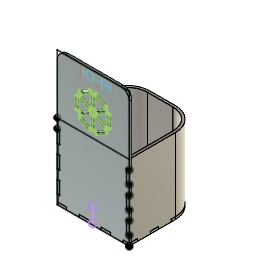
porta_lapices_v1 (Autodesk Fusion 360 design; units mm, degrees)
Autodesk Fusion 360 part; units mm, degrees
(part 1 of 3)
sketch "Boceto1" plane through (0, 0, 0) normal (0, 0, 1) x (1, 0, 0)
  line L0 (15, 40) -> (-15, 40)
  line L1 (-40, 15) -> (-40, -40)
  line L2 (40, -40) -> (40, 15)
  line L3 (40, 40) -> (-40, -40) construction
  line L4 (-40, 40) -> (40, -40) construction
  arc A0 (-15, 40) -> (-40, 15) centre (-15, 15) ccw
  line L5 (43, -40) -> (43, 15)
  line L6 (15, 43) -> (-15, 43)
  arc A1 (-15, 43) -> (-43, 15) centre (-15, 15) ccw
  line L7 (-43, 15) -> (-43, -40)
  line L8 (-40, -40) -> (-43, -40)
  line L9 (40, -40) -> (43, -40)
  arc A2 (40, 15) -> (15, 40) centre (15, 15) ccw
  arc A3 (43, 15) -> (15, 43) centre (15, 15) ccw
  dimension "d1" = 80
  dimension "d2" = 80
  dimension "d3" = 25
  dimension "d32" = 25
  dimension "d33" = 28
  constraint horizontal L0
  constraint perpendicular L0 L1
  constraint parallel L1 L2
  constraint coincident L3 origin
  constraint coincident L4 origin
  constraint coincident L4.start L1
  constraint coincident L4.start L0
  constraint tangent L1 A0
  constraint tangent L0 A0
  constraint coincident L3.start L0
  constraint coincident L3.start L2
  constraint perpendicular L7 L8
  constraint perpendicular L5 L9
  constraint concentric A0 A1
  constraint tangent A1 L7
  constraint tangent L6 A1
  constraint coincident L6 A1.end
  constraint tangent L2 A2
  constraint tangent L0 A2
  constraint tangent L5 A3
  constraint tangent L6 A3
  measures "d1" distance of L1.end L2.start
  measures "d2" distance of L4.start L1.end
  measures "d3" radius of A0
  measures "d32" radius of A2
  measures "d33" radius of A3
extrude "Extruir1" add sketch "Boceto1" along normal blind 90 makes body 1
sketch "Boceto5" plane through (0, -40, 0) normal (0, -1, 0) x (1, 0, 0)
  line L0 (-43, 0) -> (-40, 0)
  line L1 (-40, 0) -> (-40, 90)
  line L2 (-40, 90) -> (-43, 90)
  line L3 (-43, 90) -> (-43, 0)
  line L4 (-43, 90) -> (43, 90)
  line L5 (43, 90) -> (43, 0)
  line L6 (43, 0) -> (-43, 0)
  line L7 (-43, 0) -> (-43, 90)
  line L8 (-43, 78.75) -> (-40, 78.75)
  line L9 (-40, 78.75) -> (-40, 63.75)
  line L10 (-40, 63.75) -> (-43, 63.75)
  line L11 (-43, 63.75) -> (-43, 78.75)
  line L12 (-43, 52.5) -> (-40, 52.5)
  line L13 (-40, 52.5) -> (-40, 37.5)
  line L14 (-40, 37.5) -> (-43, 37.5)
  line L15 (-43, 37.5) -> (-43, 52.5)
  line L16 (-43, 26.25) -> (-40, 26.25)
  line L17 (-40, 26.25) -> (-40, 11.25)
  line L18 (-40, 11.25) -> (-43, 11.25)
  line L19 (-43, 11.25) -> (-43, 26.25)
  line L20 (-41.5, 78.75) -> (-41.5, 90) construction
  line L21 (-41.5, 63.75) -> (-41.5, 52.5) construction
  line L22 (-41.5, 37.5) -> (-41.5, 26.25) construction
  line L23 (-41.5, 11.25) -> (-41.5, 0) construction
  line L24 (0, 20) -> (0, 2.5)
  line L25 (43, 78.75) -> (40, 78.75)
  line L26 (40, 78.75) -> (40, 63.75)
  line L27 (40, 63.75) -> (43, 63.75)
  line L28 (40, 52.5) -> (40, 37.5)
  line L29 (43, 52.5) -> (40, 52.5)
  line L30 (40, 37.5) -> (43, 37.5)
  line L31 (43, 26.25) -> (40, 26.25)
  line L32 (40, 26.25) -> (40, 11.25)
  line L33 (40, 11.25) -> (43, 11.25)
  line L34 (-43, 160) -> (43, 160)
  line L35 (43, 160) -> (43, 90)
  line L36 (-43, 90) -> (-43, 160)
  line L37 (-4.7613, 96.0744) -> (-4.9442, 96.1341)
  line L38 (-4.9442, 96.1341) -> (-5.0659, 96.2025)
  spline S0 degree 3 poles (-5.0659, 96.2025) (-5.1328, 96.2402) (-7.6163, 97.6743) (-10.5848, 99.3893) knots 0 0 0 0 1 1 1 1
  line L39 (-10.5848, 99.3893) -> (-15.9822, 102.5077)
  line L40 (-15.9822, 102.5077) -> (-16.0924, 102.5916)
  spline S1 degree 3 poles (-16.0924, 102.5916) (-16.153, 102.6377) (-16.2592, 102.7361) (-16.3285, 102.8101) knots 0 0 0 0 1 1 1 1
  line L41 (-16.3285, 102.8101) -> (-16.4544, 102.9447)
  line L42 (-16.4544, 102.9447) -> (-16.5495, 103.1069)
  line L43 (-16.5495, 103.1069) -> (-16.6447, 103.269)
  line L44 (-16.6447, 103.269) -> (-16.7101, 103.4685)
  line L45 (-16.7101, 103.4685) -> (-16.7754, 103.6681)
  line L46 (-16.7754, 103.6681) -> (-16.785, 103.9516)
  line L47 (-16.785, 103.9516) -> (-16.7946, 104.2351)
  line L48 (-16.7946, 104.2351) -> (-16.7633, 104.3825)
  spline S2 degree 3 poles (-16.7633, 104.3825) (-16.7461, 104.4635) (-16.7028, 104.6053) (-16.6672, 104.6975) knots 0 0 0 0 1 1 1 1
  line L49 (-16.6672, 104.6975) -> (-16.6024, 104.8651)
  line L50 (-16.6024, 104.8651) -> (-16.5142, 104.9997)
  spline S3 degree 3 poles (-16.5142, 104.9997) (-16.4658, 105.0737) (-16.3697, 105.1945) (-16.3008, 105.2682) knots 0 0 0 0 1 1 1 1
  line L51 (-16.3008, 105.2682) -> (-16.1755, 105.4021)
  line L52 (-16.1755, 105.4021) -> (-15.999, 105.5196)
  line L53 (-15.999, 105.5196) -> (-15.8224, 105.637)
  line L54 (-15.8224, 105.637) -> (-15.6713, 105.6957)
  line L55 (-15.6713, 105.6957) -> (-15.5201, 105.7543)
  line L56 (-15.5201, 105.7543) -> (-15.343, 105.7902)
  line L57 (-15.343, 105.7902) -> (-15.1659, 105.8261)
  line L58 (-15.1659, 105.8261) -> (-14.9125, 105.8147)
  line L59 (-14.9125, 105.8147) -> (-14.6591, 105.8034)
  line L60 (-14.6591, 105.8034) -> (-14.5052, 105.759)
  line L61 (-14.5052, 105.759) -> (-14.3513, 105.7146)
  line L62 (-14.3513, 105.7146) -> (-14.2217, 105.6493)
  spline S4 degree 3 poles (-14.2217, 105.6493) (-14.1504, 105.6134) (-11.6538, 104.1758) (-8.6737, 102.4548) knots 0 0 0 0 1 1 1 1
  line L63 (-8.6737, 102.4548) -> (-3.2554, 99.3256)
  line L64 (-3.2554, 99.3256) -> (-3.0994, 99.2079)
  line L65 (-3.0994, 99.2079) -> (-2.9434, 99.0901)
  line L66 (-2.9434, 99.0901) -> (-2.8301, 98.9534)
  spline S5 degree 3 poles (-2.8301, 98.9534) (-2.6895, 98.7838) (-2.5801, 98.5915) (-2.5074, 98.3861) knots 0 0 0 0 1 1 1 1
  line L67 (-2.5074, 98.3861) -> (-2.4515, 98.2285)
  line L68 (-2.4515, 98.2285) -> (-2.4252, 98.0654)
  line L69 (-2.4252, 98.0654) -> (-2.3989, 97.9023)
  line L70 (-2.3989, 97.9023) -> (-2.4109, 97.677)
  line L71 (-2.4109, 97.677) -> (-2.4228, 97.4517)
  line L72 (-2.4228, 97.4517) -> (-2.4668, 97.298)
  line L73 (-2.4668, 97.298) -> (-2.5107, 97.1444)
  line L74 (-2.5107, 97.1444) -> (-2.5919, 96.983)
  line L75 (-2.5919, 96.983) -> (-2.6731, 96.8216)
  line L76 (-2.6731, 96.8216) -> (-2.7709, 96.6914)
  spline S6 degree 3 poles (-2.7709, 96.6914) (-2.9905, 96.3994) (-3.3229, 96.1708) (-3.6934, 96.0572) knots 0 0 0 0 1 1 1 1
  line L77 (-3.6934, 96.0572) -> (-3.8373, 96.0131)
  line L78 (-3.8373, 96.0131) -> (-4.2079, 96.0139)
  line L79 (-4.2079, 96.0139) -> (-4.5785, 96.0147)
  line L80 (-4.5785, 96.0147) -> (-4.7613, 96.0744)
  spline S7 degree 3 poles (-3.947, 96.0562) (-3.6813, 96.1032) (-3.4436, 96.2003) (-3.2159, 96.3547) knots 0 0 0 0 1 1 1 1
  line L81 (-3.2159, 96.3547) -> (-3.0924, 96.4384)
  line L82 (-3.0924, 96.4384) -> (-2.9655, 96.567)
  line L83 (-2.9655, 96.567) -> (-2.8386, 96.6956)
  line L84 (-2.8386, 96.6956) -> (-2.7384, 96.8488)
  line L85 (-2.7384, 96.8488) -> (-2.6382, 97.0019)
  line L86 (-2.6382, 97.0019) -> (-2.5742, 97.1678)
  line L87 (-2.5742, 97.1678) -> (-2.5102, 97.3337)
  line L88 (-2.5102, 97.3337) -> (-2.4764, 97.5292)
  line L89 (-2.4764, 97.5292) -> (-2.4425, 97.7247)
  line L90 (-2.4425, 97.7247) -> (-2.4568, 97.8898)
  line L91 (-2.4568, 97.8898) -> (-2.4711, 98.0549)
  line L92 (-2.4711, 98.0549) -> (-2.5105, 98.2052)
  spline S8 degree 3 poles (-2.5105, 98.2052) (-2.6122, 98.5936) (-2.8445, 98.9405) (-3.1621, 99.1785) knots 0 0 0 0 1 1 1 1
  line L93 (-3.1621, 99.1785) -> (-3.2764, 99.2641)
  line L94 (-3.2764, 99.2641) -> (-8.7367, 102.4202)
  line L95 (-8.7367, 102.4202) -> (-14.1971, 105.5763)
  line L96 (-14.1971, 105.5763) -> (-14.3653, 105.6451)
  line L97 (-14.3653, 105.6451) -> (-14.5336, 105.714)
  line L98 (-14.5336, 105.714) -> (-14.7328, 105.7486)
  line L99 (-14.7328, 105.7486) -> (-14.9321, 105.7832)
  line L100 (-14.9321, 105.7832) -> (-15.1074, 105.7692)
  line L101 (-15.1074, 105.7692) -> (-15.2826, 105.7552)
  line L102 (-15.2826, 105.7552) -> (-15.4644, 105.7025)
  line L103 (-15.4644, 105.7025) -> (-15.6461, 105.6499)
  line L104 (-15.6461, 105.6499) -> (-15.8042, 105.5658)
  line L105 (-15.8042, 105.5658) -> (-15.9623, 105.4816)
  line L106 (-15.9623, 105.4816) -> (-16.0977, 105.3723)
  line L107 (-16.0977, 105.3723) -> (-16.2331, 105.2631)
  line L108 (-16.2331, 105.2631) -> (-16.3447, 105.1271)
  line L109 (-16.3447, 105.1271) -> (-16.4563, 104.9911)
  line L110 (-16.4563, 104.9911) -> (-16.5586, 104.7811)
  line L111 (-16.5586, 104.7811) -> (-16.661, 104.5711)
  line L112 (-16.661, 104.5711) -> (-16.6955, 104.4346)
  line L113 (-16.6955, 104.4346) -> (-16.73, 104.2981)
  line L114 (-16.73, 104.2981) -> (-16.7415, 104.0986)
  line L115 (-16.7415, 104.0986) -> (-16.753, 103.8991)
  line L116 (-16.753, 103.8991) -> (-16.7101, 103.692)
  line L117 (-16.7101, 103.692) -> (-16.6671, 103.485)
  line L118 (-16.6671, 103.485) -> (-16.5626, 103.272)
  line L119 (-16.5626, 103.272) -> (-16.458, 103.059)
  line L120 (-16.458, 103.059) -> (-16.3418, 102.919)
  line L121 (-16.3418, 102.919) -> (-16.2256, 102.779)
  line L122 (-16.2256, 102.779) -> (-16.0999, 102.6775)
  line L123 (-16.0999, 102.6775) -> (-15.9743, 102.576)
  line L124 (-15.9743, 102.576) -> (-10.5599, 99.4468)
  spline S9 degree 3 poles (-10.5599, 99.4468) (-7.5821, 97.7257) (-5.0794, 96.283) (-4.9985, 96.2406) knots 0 0 0 0 1 1 1 1
  spline S10 degree 3 poles (-4.9985, 96.2406) (-4.7337, 96.102) (-4.502, 96.0412) (-4.22, 96.0365) knots 0 0 0 0 1 1 1 1
  line L125 (-4.22, 96.0365) -> (-4.0716, 96.0341)
  line L126 (-4.0716, 96.0341) -> (-3.947, 96.0562)
  line L127 (3.3017, 96.0749) -> (3.1173, 96.135)
  line L128 (3.1173, 96.135) -> (2.9557, 96.2263)
  line L129 (2.9557, 96.2263) -> (2.7942, 96.3176)
  line L130 (2.7942, 96.3176) -> (2.6046, 96.5066)
  line L131 (2.6046, 96.5066) -> (2.415, 96.6956)
  line L132 (2.415, 96.6956) -> (2.3161, 96.8636)
  line L133 (2.3161, 96.8636) -> (2.2172, 97.0316)
  line L134 (2.2172, 97.0316) -> (2.1502, 97.2312)
  line L135 (2.1502, 97.2312) -> (2.0831, 97.4307)
  line L136 (2.0831, 97.4307) -> (2.0732, 97.7039)
  line L137 (2.0732, 97.7039) -> (2.0633, 97.9772)
  line L138 (2.0633, 97.9772) -> (2.0972, 98.1409)
  line L139 (2.0972, 98.1409) -> (2.131, 98.3047)
  line L140 (2.131, 98.3047) -> (2.1942, 98.4625)
  line L141 (2.1942, 98.4625) -> (2.2574, 98.6203)
  line L142 (2.2574, 98.6203) -> (2.3547, 98.7711)
  line L143 (2.3547, 98.7711) -> (2.4519, 98.9218)
  line L144 (2.4519, 98.9218) -> (2.6014, 99.0693)
  line L145 (2.6014, 99.0693) -> (2.751, 99.2168)
  line L146 (2.751, 99.2168) -> (2.9085, 99.3138)
  spline S11 degree 3 poles (2.9085, 99.3138) (3.1847, 99.484) (13.7289, 105.5719) (13.873, 105.6444) knots 0 0 0 0 1 1 1 1
  line L147 (13.873, 105.6444) -> (14.0113, 105.7139)
  line L148 (14.0113, 105.7139) -> (14.1775, 105.7619)
  line L149 (14.1775, 105.7619) -> (14.3437, 105.81)
  line L150 (14.3437, 105.81) -> (14.6587, 105.81)
  line L151 (14.6587, 105.81) -> (14.9738, 105.81)
  line L152 (14.9738, 105.81) -> (15.1373, 105.7627)
  line L153 (15.1373, 105.7627) -> (15.3008, 105.7154)
  line L154 (15.3008, 105.7154) -> (15.4628, 105.6339)
  line L155 (15.4628, 105.6339) -> (15.6248, 105.5525)
  line L156 (15.6248, 105.5525) -> (15.7558, 105.454)
  line L157 (15.7558, 105.454) -> (15.8867, 105.3555)
  line L158 (15.8867, 105.3555) -> (15.9934, 105.2363)
  spline S12 degree 3 poles (15.9934, 105.2363) (16.0521, 105.1708) (16.1423, 105.0499) (16.1937, 104.9676) knots 0 0 0 0 1 1 1 1
  line L159 (16.1937, 104.9676) -> (16.2873, 104.8181)
  line L160 (16.2873, 104.8181) -> (16.3475, 104.6526)
  line L161 (16.3475, 104.6526) -> (16.4078, 104.4871)
  line L162 (16.4078, 104.4871) -> (16.434, 104.3241)
  line L163 (16.434, 104.3241) -> (16.4602, 104.1611)
  line L164 (16.4602, 104.1611) -> (16.4484, 103.9251)
  line L165 (16.4484, 103.9251) -> (16.4366, 103.6891)
  line L166 (16.4366, 103.6891) -> (16.3916, 103.5324)
  line L167 (16.3916, 103.5324) -> (16.3467, 103.3757)
  line L168 (16.3467, 103.3757) -> (16.2535, 103.1951)
  line L169 (16.2535, 103.1951) -> (16.1602, 103.0146)
  line L170 (16.1602, 103.0146) -> (16.0458, 102.8758)
  line L171 (16.0458, 102.8758) -> (15.9313, 102.737)
  line L172 (15.9313, 102.737) -> (15.8039, 102.634)
  line L173 (15.8039, 102.634) -> (15.6766, 102.531)
  line L174 (15.6766, 102.531) -> (10.219, 99.3771)
  spline S13 degree 3 poles (10.219, 99.3771) (7.2173, 97.6425) (4.7059, 96.1959) (4.6382, 96.1625) knots 0 0 0 0 1 1 1 1
  spline S14 degree 3 poles (4.6382, 96.1625) (4.5705, 96.129) (4.4503, 96.0817) (4.3711, 96.0573) knots 0 0 0 0 1 1 1 1
  line L175 (4.3711, 96.0573) -> (4.2272, 96.0131)
  line L176 (4.2272, 96.0131) -> (3.8566, 96.0139)
  line L177 (3.8566, 96.0139) -> (3.486, 96.0147)
  line L178 (3.486, 96.0147) -> (3.3017, 96.0749)
  spline S15 degree 3 poles (4.2618, 96.0858) (4.3304, 96.1044) (4.4401, 96.1413) (4.5056, 96.1677) knots 0 0 0 0 1 1 1 1
  line L179 (4.5056, 96.1677) -> (4.6247, 96.2158)
  line L180 (4.6247, 96.2158) -> (10.0722, 99.3629)
  spline S16 degree 3 poles (10.0722, 99.3629) (13.0684, 101.0939) (15.5752, 102.5473) (15.643, 102.5927) knots 0 0 0 0 1 1 1 1
  line L181 (15.643, 102.5927) -> (15.7662, 102.6754)
  line L182 (15.7662, 102.6754) -> (15.891, 102.8002)
  line L183 (15.891, 102.8002) -> (16.0158, 102.925)
  line L184 (16.0158, 102.925) -> (16.1184, 103.0821)
  line L185 (16.1184, 103.0821) -> (16.2209, 103.2393)
  line L186 (16.2209, 103.2393) -> (16.2849, 103.4052)
  line L187 (16.2849, 103.4052) -> (16.3489, 103.5711)
  line L188 (16.3489, 103.5711) -> (16.3829, 103.7666)
  line L189 (16.3829, 103.7666) -> (16.4168, 103.9621)
  line L190 (16.4168, 103.9621) -> (16.4028, 104.1373)
  line L191 (16.4028, 104.1373) -> (16.3888, 104.3126)
  line L192 (16.3888, 104.3126) -> (16.3363, 104.4943)
  line L193 (16.3363, 104.4943) -> (16.2839, 104.6761)
  line L194 (16.2839, 104.6761) -> (16.1995, 104.8328)
  line L195 (16.1995, 104.8328) -> (16.1152, 104.9895)
  line L196 (16.1152, 104.9895) -> (16.0086, 105.121)
  spline S17 degree 3 poles (16.0086, 105.121) (15.8856, 105.2726) (15.7612, 105.3819) (15.5741, 105.5029) knots 0 0 0 0 1 1 1 1
  line L197 (15.5741, 105.5029) -> (15.4418, 105.5883)
  line L198 (15.4418, 105.5883) -> (15.2773, 105.6518)
  line L199 (15.2773, 105.6518) -> (15.1127, 105.7153)
  line L200 (15.1127, 105.7153) -> (14.9172, 105.7492)
  line L201 (14.9172, 105.7492) -> (14.7217, 105.7832)
  line L202 (14.7217, 105.7832) -> (14.5465, 105.7692)
  line L203 (14.5465, 105.7692) -> (14.3712, 105.7552)
  line L204 (14.3712, 105.7552) -> (14.1932, 105.7036)
  spline S18 degree 3 poles (14.1932, 105.7036) (14.0953, 105.6752) (13.9757, 105.632) (13.9274, 105.6075) knots 0 0 0 0 1 1 1 1
  spline S19 degree 3 poles (13.9274, 105.6075) (13.7892, 105.5374) (3.0607, 99.3373) (2.9105, 99.2406) knots 0 0 0 0 1 1 1 1
  line L205 (2.9105, 99.2406) -> (2.776, 99.1541)
  line L206 (2.776, 99.1541) -> (2.6464, 99.0264)
  line L207 (2.6464, 99.0264) -> (2.5167, 98.8986)
  line L208 (2.5167, 98.8986) -> (2.432, 98.7737)
  spline S20 degree 3 poles (2.432, 98.7737) (2.3086, 98.5917) (2.2438, 98.4542) (2.1837, 98.2468) knots 0 0 0 0 1 1 1 1
  line L209 (2.1837, 98.2468) -> (2.1304, 98.0629)
  line L210 (2.1304, 98.0629) -> (2.1176, 97.8832)
  line L211 (2.1176, 97.8832) -> (2.1049, 97.7036)
  line L212 (2.1049, 97.7036) -> (2.1313, 97.5461)
  line L213 (2.1313, 97.5461) -> (2.1576, 97.3887)
  line L214 (2.1576, 97.3887) -> (2.2132, 97.2312)
  spline S21 degree 3 poles (2.2132, 97.2312) (2.2806, 97.0402) (2.3908, 96.8417) (2.5188, 96.6805) knots 0 0 0 0 1 1 1 1
  line L215 (2.5188, 96.6805) -> (2.6142, 96.5603)
  line L216 (2.6142, 96.5603) -> (2.7542, 96.4448)
  line L217 (2.7542, 96.4448) -> (2.8943, 96.3293)
  line L218 (2.8943, 96.3293) -> (3.0536, 96.2468)
  spline S22 degree 3 poles (3.0536, 96.2468) (3.2371, 96.152) (3.3668, 96.1052) (3.5595, 96.0642) knots 0 0 0 0 1 1 1 1
  line L219 (3.5595, 96.0642) -> (3.696, 96.0353)
  line L220 (3.696, 96.0353) -> (3.9166, 96.0436)
  line L221 (3.9166, 96.0436) -> (4.1371, 96.052)
  line L222 (4.1371, 96.052) -> (4.2618, 96.0858)
  spline S23 degree 3 poles (-0.3677, 98.3158) (-0.3966, 98.3202) (-0.4769, 98.3339) (-0.5462, 98.3464) knots 0 0 0 0 1 1 1 1
  line L223 (-0.5462, 98.3464) -> (-0.6722, 98.3691)
  line L224 (-0.6722, 98.3691) -> (-0.8328, 98.4308)
  line L225 (-0.8328, 98.4308) -> (-0.9933, 98.4926)
  line L226 (-0.9933, 98.4926) -> (-1.1268, 98.5788)
  spline S24 degree 3 poles (-1.1268, 98.5788) (-1.2002, 98.6262) (-1.3095, 98.7071) (-1.3697, 98.7585) knots 0 0 0 0 1 1 1 1
  line L227 (-1.3697, 98.7585) -> (-1.4792, 98.852)
  line L228 (-1.4792, 98.852) -> (-1.5941, 99.0024)
  line L229 (-1.5941, 99.0024) -> (-1.7091, 99.1528)
  line L230 (-1.7091, 99.1528) -> (-1.794, 99.3313)
  line L231 (-1.794, 99.3313) -> (-1.8789, 99.5098)
  line L232 (-1.8789, 99.5098) -> (-1.9161, 99.6463)
  line L233 (-1.9161, 99.6463) -> (-1.9533, 99.7828)
  line L234 (-1.9533, 99.7828) -> (-1.9533, 106.3562)
  line L235 (-1.9533, 106.3562) -> (-1.9533, 112.9296)
  line L236 (-1.9533, 112.9296) -> (-1.8855, 113.1291)
  line L237 (-1.8855, 113.1291) -> (-1.8178, 113.3287)
  line L238 (-1.8178, 113.3287) -> (-1.7199, 113.4967)
  line L239 (-1.7199, 113.4967) -> (-1.6221, 113.6647)
  line L240 (-1.6221, 113.6647) -> (-1.4307, 113.8537)
  line L241 (-1.4307, 113.8537) -> (-1.2393, 114.0427)
  line L242 (-1.2393, 114.0427) -> (-1.0777, 114.1336)
  line L243 (-1.0777, 114.1336) -> (-0.9162, 114.2246)
  line L244 (-0.9162, 114.2246) -> (-0.7675, 114.2748)
  spline S25 degree 3 poles (-0.7675, 114.2748) (-0.6858, 114.3025) (-0.5563, 114.336) (-0.4798, 114.3494) knots 0 0 0 0 1 1 1 1
  line L245 (-0.4798, 114.3494) -> (-0.3407, 114.3736)
  line L246 (-0.3407, 114.3736) -> (-0.0759, 114.3635)
  line L247 (-0.0759, 114.3635) -> (0.1888, 114.3534)
  line L248 (0.1888, 114.3534) -> (0.3883, 114.2862)
  line L249 (0.3883, 114.2862) -> (0.5879, 114.2191)
  line L250 (0.5879, 114.2191) -> (0.7268, 114.1369)
  spline S26 degree 3 poles (0.7268, 114.1369) (0.8032, 114.0917) (0.9196, 114.0108) (0.9855, 113.9571) knots 0 0 0 0 1 1 1 1
  line L251 (0.9855, 113.9571) -> (1.1054, 113.8595)
  line L252 (1.1054, 113.8595) -> (1.2193, 113.7213)
  line L253 (1.2193, 113.7213) -> (1.3333, 113.5831)
  line L254 (1.3333, 113.5831) -> (1.4269, 113.4019)
  line L255 (1.4269, 113.4019) -> (1.5204, 113.2208)
  line L256 (1.5204, 113.2208) -> (1.5687, 113.0542)
  line L257 (1.5687, 113.0542) -> (1.6169, 112.8876)
  line L258 (1.6169, 112.8876) -> (1.6169, 106.3457)
  line L259 (1.6169, 106.3457) -> (1.6169, 99.8038)
  line L260 (1.6169, 99.8038) -> (1.5799, 99.6699)
  spline S27 degree 3 poles (1.5799, 99.6699) (1.5296, 99.4879) (1.4568, 99.3119) (1.3724, 99.1683) knots 0 0 0 0 1 1 1 1
  line L261 (1.3724, 99.1683) -> (1.3019, 99.0485)
  line L262 (1.3019, 99.0485) -> (1.1024, 98.8464)
  line L263 (1.1024, 98.8464) -> (0.9029, 98.6443)
  line L264 (0.9029, 98.6443) -> (0.7559, 98.5596)
  line L265 (0.7559, 98.5596) -> (0.6089, 98.4748)
  line L266 (0.6089, 98.4748) -> (0.4254, 98.4102)
  line L267 (0.4254, 98.4102) -> (0.2419, 98.3456)
  line L268 (0.2419, 98.3456) -> (0.0689, 98.3239)
  spline S28 degree 3 poles (0.0689, 98.3239) (-0.0995, 98.3028) (-0.261, 98.2998) (-0.3677, 98.3158) knots 0 0 0 0 1 1 1 1
  line L269 (0.2165, 98.4074) -> (0.3912, 98.4493)
  line L270 (0.3912, 98.4493) -> (0.5457, 98.5207)
  spline S29 degree 3 poles (0.5457, 98.5207) (0.7389, 98.6099) (0.8685, 98.698) (1.0261, 98.8471) knots 0 0 0 0 1 1 1 1
  line L271 (1.0261, 98.8471) -> (1.1493, 98.9638)
  line L272 (1.1493, 98.9638) -> (1.2418, 99.0931)
  line L273 (1.2418, 99.0931) -> (1.3343, 99.2224)
  line L274 (1.3343, 99.2224) -> (1.4153, 99.3976)
  line L275 (1.4153, 99.3976) -> (1.4963, 99.5728)
  line L276 (1.4963, 99.5728) -> (1.5356, 99.7303)
  line L277 (1.5356, 99.7303) -> (1.5749, 99.8878)
  line L278 (1.5749, 99.8878) -> (1.5749, 106.3247)
  line L279 (1.5749, 106.3247) -> (1.5749, 112.7616)
  line L280 (1.5749, 112.7616) -> (1.5467, 112.8981)
  spline S30 degree 3 poles (1.5467, 112.8981) (1.5312, 112.9732) (1.4908, 113.1069) (1.4568, 113.1952) knots 0 0 0 0 1 1 1 1
  line L281 (1.4568, 113.1952) -> (1.3951, 113.3557)
  line L282 (1.3951, 113.3557) -> (1.3096, 113.488)
  spline S31 degree 3 poles (1.3096, 113.488) (1.1875, 113.6768) (1.0688, 113.8118) (0.9223, 113.9284) knots 0 0 0 0 1 1 1 1
  line L283 (0.9223, 113.9284) -> (0.7947, 114.03)
  line L284 (0.7947, 114.03) -> (0.6388, 114.1128)
  spline S32 degree 3 poles (0.6388, 114.1128) (0.3776, 114.2514) (0.0876, 114.326) (-0.1892, 114.3258) knots 0 0 0 0 1 1 1 1
  line L285 (-0.1892, 114.3258) -> (-0.3152, 114.3255)
  line L286 (-0.3152, 114.3255) -> (-0.5147, 114.2847)
  line L287 (-0.5147, 114.2847) -> (-0.7142, 114.2438)
  line L288 (-0.7142, 114.2438) -> (-0.9242, 114.139)
  line L289 (-0.9242, 114.139) -> (-1.1342, 114.0343)
  line L290 (-1.1342, 114.0343) -> (-1.2665, 113.9265)
  line L291 (-1.2665, 113.9265) -> (-1.3987, 113.8186)
  line L292 (-1.3987, 113.8186) -> (-1.5149, 113.6786)
  line L293 (-1.5149, 113.6786) -> (-1.6311, 113.5386)
  line L294 (-1.6311, 113.5386) -> (-1.7356, 113.3257)
  line L295 (-1.7356, 113.3257) -> (-1.8401, 113.1129)
  line L296 (-1.8401, 113.1129) -> (-1.8807, 112.9162)
  line L297 (-1.8807, 112.9162) -> (-1.9212, 112.7195)
  line L298 (-1.9212, 112.7195) -> (-1.9214, 106.3561)
  line L299 (-1.9214, 106.3561) -> (-1.9216, 99.9927)
  line L300 (-1.9216, 99.9927) -> (-1.8997, 99.8562)
  line L301 (-1.8997, 99.8562) -> (-1.8778, 99.7197)
  line L302 (-1.8778, 99.7197) -> (-1.8185, 99.5469)
  line L303 (-1.8185, 99.5469) -> (-1.7592, 99.374)
  line L304 (-1.7592, 99.374) -> (-1.6701, 99.2241)
  line L305 (-1.6701, 99.2241) -> (-1.5811, 99.0742)
  line L306 (-1.5811, 99.0742) -> (-1.4312, 98.9164)
  line L307 (-1.4312, 98.9164) -> (-1.2813, 98.7586)
  line L308 (-1.2813, 98.7586) -> (-1.1658, 98.6802)
  spline S33 degree 3 poles (-1.1658, 98.6802) (-0.9532, 98.536) (-0.711, 98.4309) (-0.4922, 98.3879) knots 0 0 0 0 1 1 1 1
  line L309 (-0.4922, 98.3879) -> (-0.3993, 98.3697)
  line L310 (-0.3993, 98.3697) -> (-0.1788, 98.3676)
  line L311 (-0.1788, 98.3676) -> (0.0417, 98.3654)
  line L312 (0.0417, 98.3654) -> (0.2165, 98.4074)
  spline S34 degree 3 poles (-15.272, 106.8919) (-15.3319, 106.9007) (-15.45, 106.9287) (-15.5345, 106.9542) knots 0 0 0 0 1 1 1 1
  line L313 (-15.5345, 106.9542) -> (-15.6882, 107.0006)
  line L314 (-15.6882, 107.0006) -> (-15.8247, 107.0723)
  spline S35 degree 3 poles (-15.8247, 107.0723) (-15.8997, 107.1118) (-16.026, 107.1928) (-16.1052, 107.2523) knots 0 0 0 0 1 1 1 1
  line L315 (-16.1052, 107.2523) -> (-16.2493, 107.3606)
  line L316 (-16.2493, 107.3606) -> (-16.373, 107.5095)
  line L317 (-16.373, 107.5095) -> (-16.4966, 107.6583)
  line L318 (-16.4966, 107.6583) -> (-16.5892, 107.8368)
  line L319 (-16.5892, 107.8368) -> (-16.6818, 108.0153)
  line L320 (-16.6818, 108.0153) -> (-16.731, 108.1728)
  line L321 (-16.731, 108.1728) -> (-16.7802, 108.3304)
  line L322 (-16.7802, 108.3304) -> (-16.7802, 108.6664)
  line L323 (-16.7802, 108.6664) -> (-16.7802, 109.0024)
  line L324 (-16.7802, 109.0024) -> (-16.7431, 109.1389)
  line L325 (-16.7431, 109.1389) -> (-16.706, 109.2754)
  line L326 (-16.706, 109.2754) -> (-16.615, 109.4644)
  line L327 (-16.615, 109.4644) -> (-16.524, 109.6534)
  line L328 (-16.524, 109.6534) -> (-16.4052, 109.8022)
  line L329 (-16.4052, 109.8022) -> (-16.2863, 109.9509)
  line L330 (-16.2863, 109.9509) -> (-16.1498, 110.0617)
  line L331 (-16.1498, 110.0617) -> (-16.0133, 110.1724)
  line L332 (-16.0133, 110.1724) -> (-10.6004, 113.2919)
  spline S36 degree 3 poles (-10.6004, 113.2919) (-7.6233, 115.0076) (-5.1213, 116.4472) (-5.0405, 116.4911) knots 0 0 0 0 1 1 1 1
  line L333 (-5.0405, 116.4911) -> (-4.8935, 116.5709)
  line L334 (-4.8935, 116.5709) -> (-4.7045, 116.6257)
  line L335 (-4.7045, 116.6257) -> (-4.5155, 116.6804)
  line L336 (-4.5155, 116.6804) -> (-4.3143, 116.6928)
  line L337 (-4.3143, 116.6928) -> (-4.1132, 116.7053)
  line L338 (-4.1132, 116.7053) -> (-3.9421, 116.6802)
  line L339 (-3.9421, 116.6802) -> (-3.771, 116.6552)
  line L340 (-3.771, 116.6552) -> (-3.624, 116.6052)
  spline S37 degree 3 poles (-3.624, 116.6052) (-3.5432, 116.5777) (-3.4128, 116.5215) (-3.3344, 116.4803) knots 0 0 0 0 1 1 1 1
  line L341 (-3.3344, 116.4803) -> (-3.1918, 116.4053)
  line L342 (-3.1918, 116.4053) -> (-3.0598, 116.2986)
  line L343 (-3.0598, 116.2986) -> (-2.9279, 116.1919)
  line L344 (-2.9279, 116.1919) -> (-2.8134, 116.0531)
  line L345 (-2.8134, 116.0531) -> (-2.6989, 115.9143)
  line L346 (-2.6989, 115.9143) -> (-2.6065, 115.7345)
  line L347 (-2.6065, 115.7345) -> (-2.5141, 115.5548)
  line L348 (-2.5141, 115.5548) -> (-2.4674, 115.4078)
  line L349 (-2.4674, 115.4078) -> (-2.4208, 115.2608)
  line L350 (-2.4208, 115.2608) -> (-2.4101, 114.9724)
  line L351 (-2.4101, 114.9724) -> (-2.3995, 114.684)
  line L352 (-2.3995, 114.684) -> (-2.445, 114.487)
  line L353 (-2.445, 114.487) -> (-2.4905, 114.29)
  line L354 (-2.4905, 114.29) -> (-2.5628, 114.1392)
  spline S38 degree 3 poles (-2.5628, 114.1392) (-2.6618, 113.9325) (-2.7435, 113.8156) (-2.9065, 113.6471) knots 0 0 0 0 1 1 1 1
  line L355 (-2.9065, 113.6471) -> (-3.0454, 113.5035)
  line L356 (-3.0454, 113.5035) -> (-3.1609, 113.4248)
  spline S39 degree 3 poles (-3.1609, 113.4248) (-3.2244, 113.3815) (-5.7335, 111.9299) (-8.7367, 110.199) knots 0 0 0 0 1 1 1 1
  line L357 (-8.7367, 110.199) -> (-14.1971, 107.052)
  line L358 (-14.1971, 107.052) -> (-14.3469, 106.9934)
  line L359 (-14.3469, 106.9934) -> (-14.4968, 106.9348)
  line L360 (-14.4968, 106.9348) -> (-14.6804, 106.9028)
  line L361 (-14.6804, 106.9028) -> (-14.8641, 106.8708)
  line L362 (-14.8641, 106.8708) -> (-15.0136, 106.8734)
  spline S40 degree 3 poles (-15.0136, 106.8734) (-15.0958, 106.8748) (-15.2121, 106.8832) (-15.272, 106.8919) knots 0 0 0 0 1 1 1 1
  line L363 (-14.5856, 106.9791) -> (-14.4281, 107.0187)
  line L364 (-14.4281, 107.0187) -> (-14.3014, 107.078)
  spline S41 degree 3 poles (-14.3014, 107.078) (-14.2318, 107.1106) (-11.7179, 108.5531) (-8.7151, 110.2835) knots 0 0 0 0 1 1 1 1
  line L365 (-8.7151, 110.2835) -> (-3.2554, 113.4298)
  line L366 (-3.2554, 113.4298) -> (-3.1368, 113.5206)
  spline S42 degree 3 poles (-3.1368, 113.5206) (-3.0715, 113.5705) (-2.9644, 113.6706) (-2.8986, 113.743) knots 0 0 0 0 1 1 1 1
  line L367 (-2.8986, 113.743) -> (-2.7791, 113.8747)
  line L368 (-2.7791, 113.8747) -> (-2.6943, 114.0169)
  line L369 (-2.6943, 114.0169) -> (-2.6095, 114.1591)
  line L370 (-2.6095, 114.1591) -> (-2.5502, 114.3319)
  line L371 (-2.5502, 114.3319) -> (-2.4909, 114.5047)
  line L372 (-2.4909, 114.5047) -> (-2.469, 114.6412)
  spline S43 degree 3 poles (-2.469, 114.6412) (-2.4006, 115.0677) (-2.504, 115.4998) (-2.7672, 115.888) knots 0 0 0 0 1 1 1 1
  line L373 (-2.7672, 115.888) -> (-2.8507, 116.0112)
  line L374 (-2.8507, 116.0112) -> (-2.9755, 116.136)
  line L375 (-2.9755, 116.136) -> (-3.1003, 116.2607)
  line L376 (-3.1003, 116.2607) -> (-3.2424, 116.3527)
  spline S44 degree 3 poles (-3.2424, 116.3527) (-3.3206, 116.4033) (-3.4405, 116.4695) (-3.509, 116.4999) knots 0 0 0 0 1 1 1 1
  line L377 (-3.509, 116.4999) -> (-3.6334, 116.5552)
  line L378 (-3.6334, 116.5552) -> (-3.8119, 116.5992)
  line L379 (-3.8119, 116.5992) -> (-3.9904, 116.6432)
  line L380 (-3.9904, 116.6432) -> (-4.2109, 116.6419)
  line L381 (-4.2109, 116.6419) -> (-4.4315, 116.6407)
  line L382 (-4.4315, 116.6407) -> (-4.5995, 116.5962)
  line L383 (-4.5995, 116.5962) -> (-4.7675, 116.5517)
  line L384 (-4.7675, 116.5517) -> (-4.9145, 116.4817)
  spline S45 degree 3 poles (-4.9145, 116.4817) (-5.0975, 116.3946) (-15.7827, 110.2419) (-15.9754, 110.1127) knots 0 0 0 0 1 1 1 1
  line L385 (-15.9754, 110.1127) -> (-16.1156, 110.0186)
  line L386 (-16.1156, 110.0186) -> (-16.2617, 109.8648)
  line L387 (-16.2617, 109.8648) -> (-16.4079, 109.7109)
  line L388 (-16.4079, 109.7109) -> (-16.497, 109.561)
  line L389 (-16.497, 109.561) -> (-16.586, 109.4111)
  line L390 (-16.586, 109.4111) -> (-16.6453, 109.2382)
  line L391 (-16.6453, 109.2382) -> (-16.7046, 109.0654)
  line L392 (-16.7046, 109.0654) -> (-16.7265, 108.9289)
  spline S46 degree 3 poles (-16.7265, 108.9289) (-16.7385, 108.8538) (-16.7485, 108.7329) (-16.7486, 108.6602) knots 0 0 0 0 1 1 1 1
  line L393 (-16.7486, 108.6602) -> (-16.7487, 108.5281)
  line L394 (-16.7487, 108.5281) -> (-16.7154, 108.3662)
  line L395 (-16.7154, 108.3662) -> (-16.682, 108.2044)
  line L396 (-16.682, 108.2044) -> (-16.6212, 108.0463)
  line L397 (-16.6212, 108.0463) -> (-16.5603, 107.8883)
  line L398 (-16.5603, 107.8883) -> (-16.4558, 107.7291)
  line L399 (-16.4558, 107.7291) -> (-16.3513, 107.5699)
  line L400 (-16.3513, 107.5699) -> (-16.1738, 107.4019)
  line L401 (-16.1738, 107.4019) -> (-15.9964, 107.234)
  line L402 (-15.9964, 107.234) -> (-15.8108, 107.1384)
  line L403 (-15.8108, 107.1384) -> (-15.6251, 107.0427)
  line L404 (-15.6251, 107.0427) -> (-15.4744, 106.9972)
  line L405 (-15.4744, 106.9972) -> (-15.3236, 106.9516)
  line L406 (-15.3236, 106.9516) -> (-15.1804, 106.9351)
  line L407 (-15.1804, 106.9351) -> (-15.0371, 106.9187)
  line L408 (-15.0371, 106.9187) -> (-14.8901, 106.9291)
  line L409 (-14.8901, 106.9291) -> (-14.7431, 106.9395)
  line L410 (-14.7431, 106.9395) -> (-14.5856, 106.9791)
  spline S47 degree 3 poles (14.3818, 106.8919) (14.2423, 106.9123) (13.9903, 106.9888) (13.8819, 107.0437) knots 0 0 0 0 1 1 1 1
  spline S48 degree 3 poles (13.8819, 107.0437) (13.8356, 107.0671) (11.3453, 108.4991) (8.3478, 110.2258) knots 0 0 0 0 1 1 1 1
  line L411 (8.3478, 110.2258) -> (2.898, 113.3653)
  line L412 (2.898, 113.3653) -> (2.7456, 113.4805)
  line L413 (2.7456, 113.4805) -> (2.5933, 113.5958)
  line L414 (2.5933, 113.5958) -> (2.4878, 113.722)
  spline S49 degree 3 poles (2.4878, 113.722) (2.4298, 113.7914) (2.3453, 113.9108) (2.3, 113.9874) knots 0 0 0 0 1 1 1 1
  line L415 (2.3, 113.9874) -> (2.2176, 114.1267)
  line L416 (2.2176, 114.1267) -> (2.1536, 114.3186)
  line L417 (2.1536, 114.3186) -> (2.0896, 114.5105)
  line L418 (2.0896, 114.5105) -> (2.07, 114.7003)
  line L419 (2.07, 114.7003) -> (2.0503, 114.8901)
  line L420 (2.0503, 114.8901) -> (2.0689, 115.0859)
  line L421 (2.0689, 115.0859) -> (2.0875, 115.2818)
  line L422 (2.0875, 115.2818) -> (2.1329, 115.4288)
  spline S50 degree 3 poles (2.1329, 115.4288) (2.1897, 115.6129) (2.2784, 115.7912) (2.394, 115.9538) knots 0 0 0 0 1 1 1 1
  line L423 (2.394, 115.9538) -> (2.4835, 116.0798)
  line L424 (2.4835, 116.0798) -> (2.6068, 116.1964)
  spline S51 degree 3 poles (2.6068, 116.1964) (2.7653, 116.3465) (2.8872, 116.429) (3.1044, 116.5332) knots 0 0 0 0 1 1 1 1
  line L425 (3.1044, 116.5332) -> (3.2797, 116.6173)
  line L426 (3.2797, 116.6173) -> (3.4879, 116.6605)
  line L427 (3.4879, 116.6605) -> (3.696, 116.7037)
  line L428 (3.696, 116.7037) -> (3.9376, 116.6923)
  line L429 (3.9376, 116.6923) -> (4.1791, 116.6808)
  line L430 (4.1791, 116.6808) -> (4.3328, 116.6371)
  line L431 (4.3328, 116.6371) -> (4.4866, 116.5934)
  line L432 (4.4866, 116.5934) -> (4.6307, 116.5208)
  spline S52 degree 3 poles (4.6307, 116.5208) (4.8613, 116.4047) (15.6356, 110.1922) (15.7428, 110.1136) knots 0 0 0 0 1 1 1 1
  spline S53 degree 3 poles (15.7428, 110.1136) (15.7961, 110.0745) (15.9016, 109.9769) (15.9771, 109.8968) knots 0 0 0 0 1 1 1 1
  line L433 (15.9771, 109.8968) -> (16.1145, 109.7512)
  line L434 (16.1145, 109.7512) -> (16.2004, 109.6066)
  line L435 (16.2004, 109.6066) -> (16.2863, 109.462)
  line L436 (16.2863, 109.462) -> (16.3471, 109.2952)
  line L437 (16.3471, 109.2952) -> (16.4078, 109.1284)
  line L438 (16.4078, 109.1284) -> (16.434, 108.9654)
  line L439 (16.434, 108.9654) -> (16.4602, 108.8024)
  line L440 (16.4602, 108.8024) -> (16.4483, 108.5664)
  line L441 (16.4483, 108.5664) -> (16.4365, 108.3303)
  line L442 (16.4365, 108.3303) -> (16.3936, 108.1858)
  spline S54 degree 3 poles (16.3936, 108.1858) (16.3384, 107.9998) (16.2485, 107.8085) (16.1438, 107.6546) knots 0 0 0 0 1 1 1 1
  line L443 (16.1438, 107.6546) -> (16.0607, 107.5323)
  line L444 (16.0607, 107.5323) -> (15.895, 107.3741)
  line L445 (15.895, 107.3741) -> (15.7293, 107.2159)
  line L446 (15.7293, 107.2159) -> (15.6026, 107.1389)
  spline S55 degree 3 poles (15.6026, 107.1389) (15.5329, 107.0966) (15.4046, 107.0334) (15.3176, 106.9986) knots 0 0 0 0 1 1 1 1
  line L447 (15.3176, 106.9986) -> (15.1594, 106.9352)
  line L448 (15.1594, 106.9352) -> (14.9746, 106.903)
  line L449 (14.9746, 106.903) -> (14.7897, 106.8708)
  line L450 (14.7897, 106.8708) -> (14.6402, 106.8734)
  spline S56 degree 3 poles (14.6402, 106.8734) (14.558, 106.8748) (14.4417, 106.8832) (14.3818, 106.8919) knots 0 0 0 0 1 1 1 1
  line L451 (15.008, 106.9658) -> (15.1472, 106.9935)
  line L452 (15.1472, 106.9935) -> (15.3104, 107.0614)
  line L453 (15.3104, 107.0614) -> (15.4735, 107.1293)
  line L454 (15.4735, 107.1293) -> (15.6249, 107.2305)
  line L455 (15.6249, 107.2305) -> (15.7763, 107.3318)
  line L456 (15.7763, 107.3318) -> (15.9106, 107.4743)
  spline S57 degree 3 poles (15.9106, 107.4743) (15.9844, 107.5526) (16.0816, 107.6722) (16.1266, 107.7401) knots 0 0 0 0 1 1 1 1
  line L457 (16.1266, 107.7401) -> (16.2083, 107.8634)
  line L458 (16.2083, 107.8634) -> (16.278, 108.0344)
  line L459 (16.278, 108.0344) -> (16.3477, 108.2054)
  line L460 (16.3477, 108.2054) -> (16.3823, 108.4044)
  line L461 (16.3823, 108.4044) -> (16.4168, 108.6034)
  line L462 (16.4168, 108.6034) -> (16.4028, 108.7786)
  line L463 (16.4028, 108.7786) -> (16.3888, 108.9539)
  line L464 (16.3888, 108.9539) -> (16.3374, 109.1312)
  line L465 (16.3374, 109.1312) -> (16.2861, 109.3085)
  line L466 (16.2861, 109.3085) -> (16.2151, 109.4495)
  spline S58 degree 3 poles (16.2151, 109.4495) (16.086, 109.7058) (15.8768, 109.9466) (15.6462, 110.1044) knots 0 0 0 0 1 1 1 1
  spline S59 degree 3 poles (15.6462, 110.1044) (15.4992, 110.205) (4.6465, 116.4518) (4.5256, 116.5054) knots 0 0 0 0 1 1 1 1
  spline S60 degree 3 poles (4.5256, 116.5054) (4.4621, 116.5336) (4.3392, 116.5755) (4.2526, 116.5985) knots 0 0 0 0 1 1 1 1
  line L467 (4.2526, 116.5985) -> (4.0951, 116.6404)
  line L468 (4.0951, 116.6404) -> (3.8536, 116.6404)
  line L469 (3.8536, 116.6404) -> (3.6121, 116.6404)
  line L470 (3.6121, 116.6404) -> (3.4452, 116.5962)
  line L471 (3.4452, 116.5962) -> (3.2783, 116.552)
  line L472 (3.2783, 116.552) -> (3.1092, 116.47)
  line L473 (3.1092, 116.47) -> (2.94, 116.3879)
  line L474 (2.94, 116.3879) -> (2.8017, 116.2831)
  spline S61 degree 3 poles (2.8017, 116.2831) (2.6357, 116.1572) (2.5152, 116.0251) (2.3869, 115.8283) knots 0 0 0 0 1 1 1 1
  line L475 (2.3869, 115.8283) -> (2.2913, 115.6818)
  line L476 (2.2913, 115.6818) -> (2.2308, 115.526)
  line L477 (2.2308, 115.526) -> (2.1703, 115.3701)
  line L478 (2.1703, 115.3701) -> (2.1404, 115.2138)
  line L479 (2.1404, 115.2138) -> (2.1105, 115.0576)
  line L480 (2.1105, 115.0576) -> (2.1105, 114.8905)
  line L481 (2.1105, 114.8905) -> (2.1105, 114.7235)
  line L482 (2.1105, 114.7235) -> (2.1437, 114.5616)
  line L483 (2.1437, 114.5616) -> (2.177, 114.3997)
  line L484 (2.177, 114.3997) -> (2.2405, 114.2466)
  line L485 (2.2405, 114.2466) -> (2.3041, 114.0935)
  line L486 (2.3041, 114.0935) -> (2.4037, 113.9421)
  line L487 (2.4037, 113.9421) -> (2.5034, 113.7907)
  line L488 (2.5034, 113.7907) -> (2.6482, 113.6524)
  spline S62 degree 3 poles (2.6482, 113.6524) (2.7278, 113.5763) (2.845, 113.4803) (2.9085, 113.4391) knots 0 0 0 0 1 1 1 1
  spline S63 degree 3 poles (2.9085, 113.4391) (3.069, 113.3348) (13.7648, 107.1737) (13.9105, 107.1015) knots 0 0 0 0 1 1 1 1
  spline S64 degree 3 poles (13.9105, 107.1015) (13.9755, 107.0693) (14.0965, 107.0224) (14.1795, 106.9973) knots 0 0 0 0 1 1 1 1
  line L489 (14.1795, 106.9973) -> (14.3302, 106.9516)
  line L490 (14.3302, 106.9516) -> (14.4735, 106.9354)
  line L491 (14.4735, 106.9354) -> (14.6167, 106.9192)
  line L492 (14.6167, 106.9192) -> (14.7427, 106.9287)
  spline S65 degree 3 poles (14.7427, 106.9287) (14.812, 106.9339) (14.9314, 106.9506) (15.008, 106.9658) knots 0 0 0 0 1 1 1 1
  spline S66 degree 3 poles (-19.2794, 109.2028) (-19.3487, 109.2135) (-19.4715, 109.2422) (-19.5524, 109.2664) knots 0 0 0 0 1 1 1 1
  line L493 (-19.5524, 109.2664) -> (-19.6994, 109.3105)
  line L494 (-19.6994, 109.3105) -> (-19.8604, 109.3958)
  line L495 (-19.8604, 109.3958) -> (-20.0214, 109.4812)
  line L496 (-20.0214, 109.4812) -> (-20.174, 109.6093)
  line L497 (-20.174, 109.6093) -> (-20.3265, 109.7374)
  line L498 (-20.3265, 109.7374) -> (-20.4394, 109.8844)
  line L499 (-20.4394, 109.8844) -> (-20.5523, 110.0315)
  line L500 (-20.5523, 110.0315) -> (-20.6337, 110.1995)
  line L501 (-20.6337, 110.1995) -> (-20.7152, 110.3675)
  line L502 (-20.7152, 110.3675) -> (-20.7481, 110.4965)
  line L503 (-20.7481, 110.4965) -> (-20.781, 110.6256)
  line L504 (-20.781, 110.6256) -> (-20.781, 117.2305)
  line L505 (-20.781, 117.2305) -> (-20.781, 123.8354)
  line L506 (-20.781, 123.8354) -> (-20.737, 123.9794)
  line L507 (-20.737, 123.9794) -> (-20.6931, 124.1233)
  line L508 (-20.6931, 124.1233) -> (-20.5953, 124.3108)
  line L509 (-20.5953, 124.3108) -> (-20.4974, 124.4984)
  line L510 (-20.4974, 124.4984) -> (-20.3324, 124.6731)
  line L511 (-20.3324, 124.6731) -> (-20.1673, 124.8479)
  line L512 (-20.1673, 124.8479) -> (-20.0152, 124.9497)
  line L513 (-20.0152, 124.9497) -> (-19.8631, 125.0514)
  line L514 (-19.8631, 125.0514) -> (-19.7077, 125.116)
  line L515 (-19.7077, 125.116) -> (-19.5524, 125.1806)
  line L516 (-19.5524, 125.1806) -> (-19.3766, 125.2162)
  line L517 (-19.3766, 125.2162) -> (-19.2009, 125.2517)
  line L518 (-19.2009, 125.2517) -> (-18.9356, 125.2413)
  line L519 (-18.9356, 125.2413) -> (-18.6703, 125.2309)
  line L520 (-18.6703, 125.2309) -> (-18.5443, 125.1968)
  line L521 (-18.5443, 125.1968) -> (-18.4183, 125.1628)
  line L522 (-18.4183, 125.1628) -> (-18.2083, 125.0593)
  line L523 (-18.2083, 125.0593) -> (-17.9983, 124.9559)
  line L524 (-17.9983, 124.9559) -> (-17.8513, 124.8315)
  line L525 (-17.8513, 124.8315) -> (-17.7043, 124.7071)
  line L526 (-17.7043, 124.7071) -> (-17.6064, 124.5822)
  spline S67 degree 3 poles (-17.6064, 124.5822) (-17.4798, 124.4204) (-17.3702, 124.2198) (-17.3069, 124.0336) knots 0 0 0 0 1 1 1 1
  line L527 (-17.3069, 124.0336) -> (-17.2563, 123.8849)
  line L528 (-17.2563, 123.8849) -> (-17.2324, 123.7311)
  line L529 (-17.2324, 123.7311) -> (-17.2085, 123.5773)
  line L530 (-17.2085, 123.5773) -> (-17.2149, 117.1194)
  line L531 (-17.2149, 117.1194) -> (-17.2212, 110.6615)
  line L532 (-17.2212, 110.6615) -> (-17.2683, 110.5104)
  spline S68 degree 3 poles (-17.2683, 110.5104) (-17.3675, 110.1912) (-17.487, 109.9828) (-17.7033, 109.7516) knots 0 0 0 0 1 1 1 1
  line L533 (-17.7033, 109.7516) -> (-17.8283, 109.618)
  line L534 (-17.8283, 109.618) -> (-17.9572, 109.526)
  spline S69 degree 3 poles (-17.9572, 109.526) (-18.028, 109.4754) (-18.1561, 109.4009) (-18.2417, 109.3603) knots 0 0 0 0 1 1 1 1
  line L535 (-18.2417, 109.3603) -> (-18.3973, 109.2866)
  line L536 (-18.3973, 109.2866) -> (-18.5653, 109.2437)
  line L537 (-18.5653, 109.2437) -> (-18.7333, 109.2009)
  line L538 (-18.7333, 109.2009) -> (-18.9434, 109.192)
  line L539 (-18.9434, 109.192) -> (-19.1534, 109.1831)
  line L540 (-19.1534, 109.1831) -> (-19.2794, 109.2028)
  line L541 (-18.4918, 109.3246) -> (-18.2923, 109.3899)
  line L542 (-18.2923, 109.3899) -> (-18.1589, 109.4691)
  spline S70 degree 3 poles (-18.1589, 109.4691) (-18.0854, 109.5126) (-17.9724, 109.591) (-17.9076, 109.6432) knots 0 0 0 0 1 1 1 1
  line L543 (-17.9076, 109.6432) -> (-17.7897, 109.7381)
  line L544 (-17.7897, 109.7381) -> (-17.6666, 109.8847)
  line L545 (-17.6666, 109.8847) -> (-17.5434, 110.0314)
  line L546 (-17.5434, 110.0314) -> (-17.4504, 110.2204)
  line L547 (-17.4504, 110.2204) -> (-17.3573, 110.4095)
  line L548 (-17.3573, 110.4095) -> (-17.3103, 110.5775)
  line L549 (-17.3103, 110.5775) -> (-17.2632, 110.7455)
  line L550 (-17.2632, 110.7455) -> (-17.257, 117.0879)
  line L551 (-17.257, 117.0879) -> (-17.2508, 123.4303)
  line L552 (-17.2508, 123.4303) -> (-17.2729, 123.6239)
  line L553 (-17.2729, 123.6239) -> (-17.295, 123.8175)
  line L554 (-17.295, 123.8175) -> (-17.3548, 123.9956)
  line L555 (-17.3548, 123.9956) -> (-17.4147, 124.1736)
  line L556 (-17.4147, 124.1736) -> (-17.5002, 124.3165)
  spline S71 degree 3 poles (-17.5002, 124.3165) (-17.5472, 124.3951) (-17.632, 124.5138) (-17.6887, 124.5803) knots 0 0 0 0 1 1 1 1
  line L557 (-17.6887, 124.5803) -> (-17.7918, 124.7012)
  line L558 (-17.7918, 124.7012) -> (-17.937, 124.8179)
  line L559 (-17.937, 124.8179) -> (-18.0823, 124.9345)
  line L560 (-18.0823, 124.9345) -> (-18.2503, 125.0161)
  line L561 (-18.2503, 125.0161) -> (-18.4183, 125.0977)
  line L562 (-18.4183, 125.0977) -> (-18.5863, 125.1453)
  line L563 (-18.5863, 125.1453) -> (-18.7543, 125.1929)
  line L564 (-18.7543, 125.1929) -> (-19.0169, 125.1928)
  line L565 (-19.0169, 125.1928) -> (-19.2794, 125.1926)
  line L566 (-19.2794, 125.1926) -> (-19.4523, 125.1441)
  line L567 (-19.4523, 125.1441) -> (-19.6252, 125.0955)
  line L568 (-19.6252, 125.0955) -> (-19.7837, 125.0144)
  line L569 (-19.7837, 125.0144) -> (-19.9422, 124.9334)
  line L570 (-19.9422, 124.9334) -> (-20.0636, 124.8399)
  spline S72 degree 3 poles (-20.0636, 124.8399) (-20.1304, 124.7885) (-20.2391, 124.6881) (-20.305, 124.6169) knots 0 0 0 0 1 1 1 1
  line L571 (-20.305, 124.6169) -> (-20.425, 124.4874)
  line L572 (-20.425, 124.4874) -> (-20.5195, 124.3263)
  line L573 (-20.5195, 124.3263) -> (-20.6139, 124.1653)
  line L574 (-20.6139, 124.1653) -> (-20.6817, 123.9658)
  line L575 (-20.6817, 123.9658) -> (-20.7495, 123.7663)
  line L576 (-20.7495, 123.7663) -> (-20.7495, 117.2349)
  line L577 (-20.7495, 117.2349) -> (-20.7495, 110.7035)
  line L578 (-20.7495, 110.7035) -> (-20.7021, 110.54)
  line L579 (-20.7021, 110.54) -> (-20.6547, 110.3765)
  line L580 (-20.6547, 110.3765) -> (-20.5725, 110.2131)
  line L581 (-20.5725, 110.2131) -> (-20.4904, 110.0497)
  line L582 (-20.4904, 110.0497) -> (-20.373, 109.9023)
  line L583 (-20.373, 109.9023) -> (-20.2556, 109.755)
  line L584 (-20.2556, 109.755) -> (-20.1245, 109.6488)
  spline S73 degree 3 poles (-20.1245, 109.6488) (-19.8952, 109.4632) (-19.6372, 109.3357) (-19.3653, 109.2738) knots 0 0 0 0 1 1 1 1
  line L585 (-19.3653, 109.2738) -> (-19.2374, 109.2446)
  line L586 (-19.2374, 109.2446) -> (-18.9643, 109.252)
  line L587 (-18.9643, 109.252) -> (-18.6913, 109.2594)
  line L588 (-18.6913, 109.2594) -> (-18.4918, 109.3246)
  spline S74 degree 3 poles (18.4165, 109.2015) (18.2257, 109.2285) (18.0587, 109.2811) (17.8747, 109.3722) knots 0 0 0 0 1 1 1 1
  spline S75 degree 3 poles (17.8747, 109.3722) (17.6551, 109.4809) (17.5384, 109.5692) (17.3538, 109.7666) knots 0 0 0 0 1 1 1 1
  line L589 (17.3538, 109.7666) -> (17.1999, 109.9311)
  line L590 (17.1999, 109.9311) -> (17.1294, 110.0489)
  spline S76 degree 3 poles (17.1294, 110.0489) (17.0504, 110.1811) (16.9782, 110.3512) (16.9224, 110.5368) knots 0 0 0 0 1 1 1 1
  line L591 (16.9224, 110.5368) -> (16.8849, 110.6615)
  line L592 (16.8849, 110.6615) -> (16.8791, 117.1509)
  line L593 (16.8791, 117.1509) -> (16.8733, 123.6403)
  line L594 (16.8733, 123.6403) -> (16.9069, 123.8083)
  line L595 (16.9069, 123.8083) -> (16.9405, 123.9763)
  line L596 (16.9405, 123.9763) -> (16.9949, 124.1128)
  spline S77 degree 3 poles (16.9949, 124.1128) (17.0248, 124.1879) (17.0876, 124.3134) (17.1344, 124.3917) knots 0 0 0 0 1 1 1 1
  line L597 (17.1344, 124.3917) -> (17.2195, 124.534)
  line L598 (17.2195, 124.534) -> (17.3527, 124.6799)
  line L599 (17.3527, 124.6799) -> (17.4859, 124.8258)
  line L600 (17.4859, 124.8258) -> (17.6702, 124.9491)
  line L601 (17.6702, 124.9491) -> (17.8545, 125.0724)
  line L602 (17.8545, 125.0724) -> (18.0353, 125.1378)
  line L603 (18.0353, 125.1378) -> (18.2161, 125.2033)
  line L604 (18.2161, 125.2033) -> (18.3568, 125.2278)
  line L605 (18.3568, 125.2278) -> (18.4975, 125.2523)
  line L606 (18.4975, 125.2523) -> (18.7622, 125.2417)
  line L607 (18.7622, 125.2417) -> (19.027, 125.2312)
  line L608 (19.027, 125.2312) -> (19.2265, 125.166)
  line L609 (19.2265, 125.166) -> (19.426, 125.1009)
  line L610 (19.426, 125.1009) -> (19.5835, 125.008)
  line L611 (19.5835, 125.008) -> (19.741, 124.9151)
  line L612 (19.741, 124.9151) -> (19.8727, 124.7953)
  spline S78 degree 3 poles (19.8727, 124.7953) (20.0305, 124.6518) (20.1631, 124.4835) (20.2626, 124.3004) knots 0 0 0 0 1 1 1 1
  line L613 (20.2626, 124.3004) -> (20.3359, 124.1653)
  line L614 (20.3359, 124.1653) -> (20.3903, 123.991)
  line L615 (20.3903, 123.991) -> (20.4446, 123.8166)
  line L616 (20.4446, 123.8166) -> (20.4446, 117.2281)
  line L617 (20.4446, 117.2281) -> (20.4446, 110.6396)
  line L618 (20.4446, 110.6396) -> (20.4021, 110.4862)
  line L619 (20.4021, 110.4862) -> (20.3595, 110.3327)
  line L620 (20.3595, 110.3327) -> (20.2942, 110.2031)
  spline S79 degree 3 poles (20.2942, 110.2031) (20.1973, 110.011) (20.0843, 109.853) (19.9415, 109.7102) knots 0 0 0 0 1 1 1 1
  line L621 (19.9415, 109.7102) -> (19.8141, 109.5829)
  line L622 (19.8141, 109.5829) -> (19.6694, 109.4867)
  spline S80 degree 3 poles (19.6694, 109.4867) (19.4905, 109.3677) (19.3374, 109.299) (19.1302, 109.2448) knots 0 0 0 0 1 1 1 1
  line L623 (19.1302, 109.2448) -> (18.9707, 109.203)
  line L624 (18.9707, 109.203) -> (18.7573, 109.1932)
  line L625 (18.7573, 109.1932) -> (18.544, 109.1835)
  line L626 (18.544, 109.1835) -> (18.4165, 109.2015)
  line L627 (19.0547, 109.2861) -> (19.2294, 109.328)
  line L628 (19.2294, 109.328) -> (19.3873, 109.4009)
  line L629 (19.3873, 109.4009) -> (19.5453, 109.4739)
  line L630 (19.5453, 109.4739) -> (19.6752, 109.5666)
  line L631 (19.6752, 109.5666) -> (19.8051, 109.6593)
  line L632 (19.8051, 109.6593) -> (19.9444, 109.807)
  line L633 (19.9444, 109.807) -> (20.0838, 109.9547)
  line L634 (20.0838, 109.9547) -> (20.1723, 110.1038)
  line L635 (20.1723, 110.1038) -> (20.2609, 110.2528)
  line L636 (20.2609, 110.2528) -> (20.3203, 110.4257)
  line L637 (20.3203, 110.4257) -> (20.3798, 110.5985)
  line L638 (20.3798, 110.5985) -> (20.4022, 110.7455)
  line L639 (20.4022, 110.7455) -> (20.4246, 110.8925)
  line L640 (20.4246, 110.8925) -> (20.4187, 117.3084)
  line L641 (20.4187, 117.3084) -> (20.4129, 123.7243)
  line L642 (20.4129, 123.7243) -> (20.3744, 123.8608)
  line L643 (20.3744, 123.8608) -> (20.3359, 123.9973)
  line L644 (20.3359, 123.9973) -> (20.2344, 124.2073)
  line L645 (20.2344, 124.2073) -> (20.1329, 124.4173)
  line L646 (20.1329, 124.4173) -> (20.0167, 124.5574)
  line L647 (20.0167, 124.5574) -> (19.9005, 124.6974)
  line L648 (19.9005, 124.6974) -> (19.7683, 124.8055)
  line L649 (19.7683, 124.8055) -> (19.636, 124.9136)
  line L650 (19.636, 124.9136) -> (19.426, 125.0155)
  line L651 (19.426, 125.0155) -> (19.216, 125.1174)
  line L652 (19.216, 125.1174) -> (19.069, 125.1548)
  line L653 (19.069, 125.1548) -> (18.922, 125.1923)
  line L654 (18.922, 125.1923) -> (18.67, 125.1923)
  line L655 (18.67, 125.1923) -> (18.418, 125.1923)
  line L656 (18.418, 125.1923) -> (18.271, 125.155)
  line L657 (18.271, 125.155) -> (18.1239, 125.1177)
  line L658 (18.1239, 125.1177) -> (17.9139, 125.0144)
  line L659 (17.9139, 125.0144) -> (17.7039, 124.9111)
  line L660 (17.7039, 124.9111) -> (17.5551, 124.7873)
  line L661 (17.5551, 124.7873) -> (17.4062, 124.6635)
  line L662 (17.4062, 124.6635) -> (17.2971, 124.5194)
  line L663 (17.2971, 124.5194) -> (17.1881, 124.3753)
  line L664 (17.1881, 124.3753) -> (17.1045, 124.2073)
  line L665 (17.1045, 124.2073) -> (17.021, 124.0393)
  line L666 (17.021, 124.0393) -> (16.9739, 123.8608)
  line L667 (16.9739, 123.8608) -> (16.9269, 123.6823)
  line L668 (16.9269, 123.6823) -> (16.9269, 117.2139)
  line L669 (16.9269, 117.2139) -> (16.9269, 110.7455)
  line L670 (16.9269, 110.7455) -> (16.9659, 110.5985)
  line L671 (16.9659, 110.5985) -> (17.005, 110.4515)
  line L672 (17.005, 110.4515) -> (17.0863, 110.2763)
  line L673 (17.0863, 110.2763) -> (17.1675, 110.101)
  line L674 (17.1675, 110.101) -> (17.26, 109.9717)
  line L675 (17.26, 109.9717) -> (17.3525, 109.8424)
  line L676 (17.3525, 109.8424) -> (17.4757, 109.7258)
  spline S81 degree 3 poles (17.4757, 109.7258) (17.6334, 109.5765) (17.7629, 109.4886) (17.9568, 109.399) knots 0 0 0 0 1 1 1 1
  line L677 (17.9568, 109.399) -> (18.112, 109.3273)
  line L678 (18.112, 109.3273) -> (18.2755, 109.2871)
  line L679 (18.2755, 109.2871) -> (18.439, 109.2469)
  line L680 (18.439, 109.2469) -> (18.6595, 109.2456)
  line L681 (18.6595, 109.2456) -> (18.88, 109.2442)
  line L682 (18.88, 109.2442) -> (19.0547, 109.2861)
  spline S82 degree 3 poles (-4.625, 117.7904) (-4.7083, 117.8128) (-4.8311, 117.8536) (-4.898, 117.8811) knots 0 0 0 0 1 1 1 1
  line L683 (-4.898, 117.8811) -> (-5.0195, 117.931)
  line L684 (-5.0195, 117.931) -> (-10.4063, 121.0347)
  spline S83 degree 3 poles (-10.4063, 121.0347) (-13.3691, 122.7417) (-15.8616, 124.1804) (-15.9452, 124.2319) knots 0 0 0 0 1 1 1 1
  line L685 (-15.9452, 124.2319) -> (-16.0973, 124.3256)
  line L686 (-16.0973, 124.3256) -> (-16.2143, 124.4325)
  spline S84 degree 3 poles (-16.2143, 124.4325) (-16.3587, 124.5645) (-16.4913, 124.7349) (-16.5877, 124.9123) knots 0 0 0 0 1 1 1 1
  line L687 (-16.5877, 124.9123) -> (-16.661, 125.0474)
  line L688 (-16.661, 125.0474) -> (-16.7196, 125.2259)
  line L689 (-16.7196, 125.2259) -> (-16.7782, 125.4044)
  line L690 (-16.7782, 125.4044) -> (-16.7789, 125.7614)
  line L691 (-16.7789, 125.7614) -> (-16.7796, 126.1185)
  line L692 (-16.7796, 126.1185) -> (-16.7122, 126.318)
  line L693 (-16.7122, 126.318) -> (-16.6447, 126.5175)
  line L694 (-16.6447, 126.5175) -> (-16.549, 126.6806)